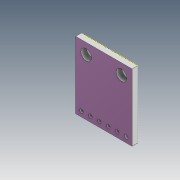
# Autodesk Inventor part: CAN_transceiver
Saved by Autodesk Inventor 2020 (Build 240168000, 168)
## iProperties
Created: 2020-09-27
Part Number: CAN_transceiver
Material: Generic
Document SubType Name: Modeling
Designer: DELL
Density: 1 g/cm^3
Appearance: Default
Author: DELL
Autodesk Inventor part; units mm, degrees
ref_plane "YZ Plane" through (0, 0, 0) normal (1, 0, 0) x (0, 1, 0)
ref_plane "XZ Plane" through (0, 0, 0) normal (0, 1, 0) x (-1, 0, 0)
ref_plane "XY Plane" through (0, 0, 0) normal (0, 0, 1) x (1, 0, 0)
sketch "Sketch1" plane through (0, 0, 0) normal (0, 0, 1) x (1, 0, 0)
  line L0 (8, -9.5) -> (-8, -9.5)
  line L1 (-8, -9.5) -> (-8, 9.5)
  line L2 (-8, 9.5) -> (8, 9.5)
  line L3 (8, 9.5) -> (8, -9.5)
  line L4 (8, -9.5) -> (-8, 9.5) construction
  line L5 (-8, -9.5) -> (8, 9.5) construction
  circle A0 centre (-5, 6.5) radius 1.5
  circle A1 centre (5, 6.5) radius 1.5
  circle A2 centre (-6.35, -8) radius 0.5
  line L6 (0, 9.5) -> (0, -9.5) construction
  circle A3 centre (-3.81, -8) radius 0.5
  circle A4 centre (-1.27, -8) radius 0.5
  circle A5 centre (1.27, -8) radius 0.5
  circle A6 centre (3.81, -8) radius 0.5
  circle A7 centre (6.35, -8) radius 0.5
  point P0 (0, 0)
  dimension "d0" = 16
  dimension "d1" = 19
  dimension "d3" = 3
  dimension "d4" = 1
  dimension "d5" = 3
  dimension "d6" = 3
  dimension "d7" = 1.5
  dimension "d10" = 2.54
  constraints: 14 end point, 8 centre point, 4 midpoint, 2 horizontal, 2 parallel, 2 symmetric about line, 1 equal radius, 1 horizontal alignment, 1 perpendicular, 10 other
  measures "d0" distance of L1.end L2.end
  measures "d1" distance of L0.end L1.end
  measures "d3" diameter of A0
  measures "d4" diameter of A2
  measures "d5" distance from line of L2 A0.centre
  measures "d6" distance from line of L1 A0.centre
  measures "d7" distance from line of L0 A2.centre
  measures "d10" distance of A2.centre A3.centre
extrude "Extrusion1" add sketch "Sketch1" along normal blind 1.6
sketch "Sketch2" plane through (0, 0, 0) normal (0, 0, -1) x (-1, 0, 0)
  line L0 (2.55, -1) -> (-2.55, -1)
  line L1 (-2.55, -1) -> (-2.55, 2.8)
  line L2 (-2.55, 2.8) -> (2.55, 2.8)
  line L3 (2.55, 2.8) -> (2.55, -1)
  line L4 (2.55, -1) -> (-2.55, 2.8) construction
  line L5 (-2.55, -1) -> (2.55, 2.8) construction
  line L6 (-8, 9.5) -> (8, 9.5) projected
  point P0 (0, 0)
  point P1 (0, 0.9)
  point P2 (0, 0.9)
  dimension "d17" = 5.1
  dimension "d18" = 3.8
  dimension "d19" = 10.5
  constraints: 12 end point, 3 midpoint, 2 parallel, 1 horizontal, 1 perpendicular, 1 vertical alignment
  measures "d17" distance of L1.end L2.end
  measures "d18" distance of L2.end L0.start
  measures "d19" distance between parallel lines of L6 L0
extrude "Extrusion2" add sketch "Sketch2" along normal blind 1.5
chamfer "Chamfer1" distance 0.3 angle 45 2 edges at (0, -1, -1.5) (0, 2.8, -1.5)
sketch "Sketch3" plane through (0, 0, 0) normal (0, 0, -1) x (-1, 0, 0)
  line L0 (-8.0252, -9.5) -> (-8.0252, 9.5) construction
  line L1 (-8.0252, 9.5) -> (7.8645, 9.5) construction
  line L2 (7.8645, 9.5) -> (7.8645, -9.5) construction
  line L3 (7.8645, -9.5) -> (-8.0252, -9.5) construction
  line L4 (8, -9.5) -> (-8, -9.5) projected
  line L5 (-8, 9.5) -> (8, 9.5) projected
  point P0 (0, 0)
  constraints: 2 collinear, 2 other
body "Solid1"
